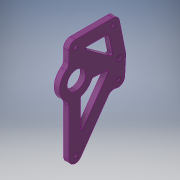
# Autodesk Inventor part: carriage plate for intake
Saved by Autodesk Inventor 2018 (Build 220112000, 112)
## iProperties
Created: 2018-01-19
Part Number: carriage plate for intake
Material: Aluminum 6061
Document SubType Name: Modeling
Designer: Ben
Density: 2.7 g/cm^3
Appearance: Smooth - Purple
Mass: 90.6899 g
Surface Area: 153.888 cm^2
Volume: 33.5889 cm^3
Author: Ben
Autodesk Inventor part; units mm, degrees
ref_plane "YZ Plane" through (0, 0, 0) normal (1, 0, 0) x (0, 1, 0)
ref_plane "XZ Plane" through (0, 0, 0) normal (0, 1, 0) x (-1, 0, 0)
ref_plane "XY Plane" through (0, 0, 0) normal (0, 0, 1) x (1, 0, 0)
sketch "Sketch1" plane through (0, 0, 0) normal (1, 0, 0) x (0, 1, 0)
  line L0 (-162.6843, 12.7) -> (420.7488, 12.7) construction
  line L1 (420.7488, 12.7) -> (420.7488, -12.7) construction
  line L2 (420.7488, -12.7) -> (-162.6843, -12.7) construction
  line L3 (-162.6843, -12.7) -> (-162.6843, 12.7) construction
  line L4 (0, 0) -> (0, -26.6192) construction
  circle A0 centre (0, -26.6192) radius 3.302
  circle A1 centre (38.1, 26.6192) radius 2.54
  circle A2 centre (-76.2, 26.6192) radius 2.54
  line L5 (38.1, 26.6192) -> (-76.2, 26.6192) construction
  line L6 (0, 0) -> (0, 26.6192) construction
  circle A3 centre (0, -26.6192) radius 15.875 construction
  circle A4 centre (38.1, 26.6192) radius 15.875 construction
  circle A5 centre (-76.2, 26.6192) radius 15.875 construction
  line L7 (0, -26.6192) -> (-76.2, 26.6192) construction
  arc A6 (46.1645, 26.6192) -> (38.1, 34.6837) centre (38.1, 26.6192) ccw
  line L8 (46.1645, 26.6192) -> (46.1645, -19.05)
  line L9 (-76.2, 26.6192) -> (-76.2, 0) construction
  line L10 (38.1, 26.6192) -> (38.1, 0) construction
  line L11 (46.1645, 0) -> (-87.2704, 0) construction
  line L12 (0, -26.6192) -> (38.1, 26.6192) construction
  line L13 (0, -26.6192) -> (0, -52.0192) construction
  line L14 (13.9446, -26.6192) -> (-16.4809, -26.6192) construction
  circle A7 centre (38.1, -19.05) radius 2.54
  line L15 (38.1, -19.05) -> (38.1, 0) construction
  arc A8 (39.6714, -26.9599) -> (46.1645, -19.05) centre (38.1, -19.05) ccw
  arc A9 (-29.845, -22.7596) -> (-22.6667, -33.4524) centre (-22.225, -25.4) ccw
  line L16 (-22.225, -12.7) -> (-22.225, -25.4) construction
  circle A10 centre (-22.225, -25.4) radius 2.54
  arc A11 (-0.4417, -34.6716) -> (1.5714, -34.5291) centre (0, -26.6192) ccw
  line L17 (39.6714, -26.9599) -> (1.5714, -34.5291)
  line L18 (-0.4417, -34.6716) -> (-22.6667, -33.4524)
  circle A12 centre (2.8575, 25.4) radius 11.1125
  arc A13 (-76.2, 34.6837) -> (-80.8188, 20.0084) centre (-76.2, 26.6192) ccw
  line L19 (-53.2165, 81.474) -> (28.2575, 0) construction
  line L20 (-80.8188, 20.0084) -> (-32.8463, -13.5084)
  arc A14 (-29.845, -22.7596) -> (-32.8463, -13.5084) centre (-37.465, -20.1193) ccw
  arc A15 (19.2986, 37.8738) -> (-13.5836, 37.8738) centre (2.8575, 25.4) ccw
  arc A16 (19.2986, 37.8738) -> (25.7233, 34.6837) centre (25.7233, 42.7482) ccw
  arc A17 (-20.0083, 34.6837) -> (-13.5836, 37.8738) centre (-20.0083, 42.7482) ccw
  line L21 (38.1, 34.6837) -> (25.7233, 34.6837)
  line L22 (-20.0083, 34.6837) -> (-76.2, 34.6837)
  point P0 (0, -42.4942)
  point P1 (-162.6843, 0)
  dimension "d3" = 31.75
  dimension "d0" = 25.4
  dimension "d1" = 6.604
  dimension "d2" = 13.9192
  dimension "d4" = 38.1
  dimension "d5" = 76.2
  dimension "d10" = 25.4
  dimension "d14" = 6.35
  dimension "d22" = 12.7
  dimension "d32" = 22.225
  dimension "d33" = 22.225
  dimension "d49" = 45
  dimension "d50" = 17.907
  dimension "d52" = 35.2425
  dimension "d55" = 5.08
  dimension "d57" = 4.7625
  dimension "d63" = 25.4
  dimension "d64" = 9.525
  constraints: 46 end point, 19 point on circle, 17 centre point, 15 tangent, 13 coincident, 11 point on line, 9 equal radius, 6 horizontal, 6 vertical, 3 parallel, 3 perpendicular, 1 collinear, 1 midpoint, 1 vertical alignment, 4 other
  measures "d0" distance of L0.end L1.end
  measures "d1" diameter of A0
  measures "d2" distance from line of L2 L4.end
  measures "d4" horizontal distance of L5.start L4.end
  measures "d5" distance from line of A2.centre L6
  measures "d10" distance of L12.start L13.end
  measures "d14" distance from line of L2 L15.start
  measures "d22" distance of L16.start L16.end
  measures "d32" distance between parallel lines of L4 L16
  measures "d33" diameter of A12
  measures "d49" angle of L19 L11
  measures "d50" distance from line of L8 L19.end
  measures "d52" horizontal distance of L15.start A12.centre
  measures "d55" diameter of A1
  measures "d57" radial gap between concentric circles of A0 A11
  measures "d63" distance from line of L11 A12.centre
  measures "d64" radial gap between concentric circles of A15 A12
extrude "Extrusion1" add sketch "Sketch1" along normal blind 6.35
sketch "Sketch3" plane through (0, 0, 0) normal (-1, 0, 0) x (0, 0, 1)
  circle A0 centre (25.4, 2.8575) radius 11.1125 construction
  circle A1 centre (-25.4, -22.225) radius 2.54 construction
  circle A2 centre (-19.05, 38.1) radius 2.54 construction
  circle A3 centre (26.6192, -76.2) radius 2.54 construction
  circle A4 centre (26.6192, 38.1) radius 2.54 construction
  circle A5 centre (-26.6192, 0) radius 3.302 construction
  arc A6 (34.6837, 38.1) -> (26.6192, 46.1645) centre (26.6192, 38.1) ccw construction
  line L0 (-19.05, 46.1645) -> (26.6192, 46.1645) construction
  arc A7 (-19.05, 46.1645) -> (-26.9599, 39.6714) centre (-19.05, 38.1) ccw construction
  line L1 (-34.5291, 1.5714) -> (-26.9599, 39.6714) construction
  arc A8 (-34.5291, 1.5714) -> (-34.6716, -0.4417) centre (-26.6192, 0) ccw construction
  line L2 (-33.4524, -22.6667) -> (-34.6716, -0.4417) construction
  arc A9 (-33.4524, -22.6667) -> (-22.7596, -29.845) centre (-25.4, -22.225) ccw construction
  arc A10 (-13.5084, -32.8463) -> (-22.7596, -29.845) centre (-20.1193, -37.465) ccw construction
  line L3 (20.0084, -80.8188) -> (-13.5084, -32.8463) construction
  arc A11 (20.0084, -80.8188) -> (34.6837, -76.2) centre (26.6192, -76.2) ccw construction
  line L4 (-26.6192, 0) -> (26.6192, 38.1) construction
  circle A12 centre (26.6192, -76.2) radius 2.54 construction
  line L5 (26.6192, 38.1) -> (26.6192, -76.2) construction
  line L6 (26.6192, -76.2) -> (-26.6192, 0) construction
  line L7 (-26.6192, 0) -> (25.4, 2.8575) construction
  line L8 (26.6192, 38.1) -> (-19.05, 38.1) construction
  line L9 (-19.05, 38.1) -> (-26.6192, 0) construction
  line L10 (-13.8374, 31.75) -> (-19.0721, 5.4011)
  line L11 (-19.0721, 5.4011) -> (17.7461, 31.75)
  line L12 (17.7461, 31.75) -> (-13.8374, 31.75)
  line L13 (1.9543, 31.75) -> (1.9543, 38.1) construction
  line L14 (-16.4548, 18.5755) -> (-22.683, 19.8129) construction
  line L15 (-14.8802, -5.7147) -> (20.2692, -56.024)
  line L16 (20.2692, -56.024) -> (20.2692, -17.132)
  circle A13 centre (25.4, 2.8575) radius 11.1125 construction
  line L17 (20.2692, -36.578) -> (26.6192, -36.578) construction
  line L18 (2.6945, -30.8694) -> (-2.5109, -34.5062) construction
  line L19 (34.6837, -20.0083) -> (34.6837, -76.2) projected
  arc A14 (37.8738, -13.5836) -> (34.6837, -20.0083) centre (42.7482, -20.0083) ccw projected
  arc A15 (37.8738, -13.5836) -> (37.8738, 19.2986) centre (25.4, 2.8575) ccw projected
  arc A16 (34.6837, 25.7233) -> (37.8738, 19.2986) centre (42.7482, 25.7233) ccw projected
  line L20 (34.6837, 38.1) -> (34.6837, 25.7233) projected
  arc A17 (6.1416, -4.56) -> (20.2692, -17.132) centre (25.4, 2.8575) ccw
  arc A18 (37.8738, -13.5836) -> (37.8738, 19.2986) centre (25.4, 2.8575) ccw projected
  line L21 (6.1416, -4.56) -> (-14.8802, -5.7147)
  line L22 (-4.3693, -5.1374) -> (-4.7176, 1.2031) construction
  point P0 (0, 0)
  dimension "d58" = 6.35
  dimension "d67" = 0
  constraints: 34 end point, 5 midpoint, 5 perpendicular, 5 point on line, 4 equal length, 3 parallel, 2 coincident, 2 horizontal, 2 point on circle, 2 vertical, 1 centre point, 1 collinear, 1 concentric
  measures "d58" distance of L13.start L13.end
  measures "d67" distance between parallel lines of L4 L11
extrude "Extrusion2" cut sketch "Sketch3" against normal through all
fillet "Fillet1" radius 1.5875 7 edges at (3.175, 31.75, -13.8374) (3.175, 31.75, 17.7461) (3.175, 5.4011, -19.0721) (3.175, -5.7147, -14.8802) (3.175, -4.56, 6.1416) (3.175, -17.132, 20.2692) (3.175, -56.024, 20.2692)
body "Solid1"
